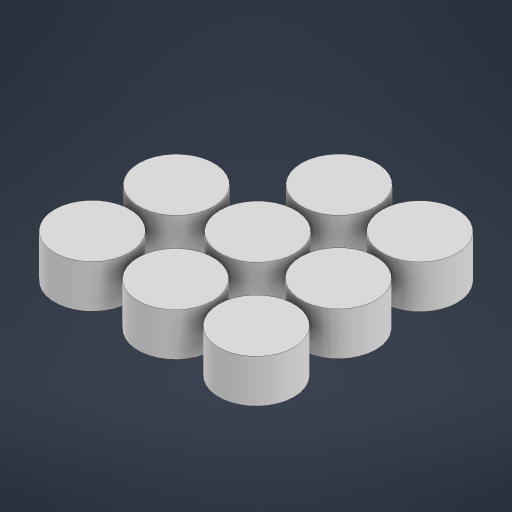
# Autodesk Inventor part: BUTTON
Saved by Autodesk Inventor 2024 (Build 280153000, 153)
## iProperties
Created: 2025-06-23
Part Number: BUTTON
Material: Generic
Document SubType Name: Modeling
Designer: ASUS
Density: 1 g/cm^3
Appearance: Default
Author: ASUS
Autodesk Inventor part; units mm, degrees
ref_plane "YZ Plane" through (0, 0, 0) normal (1, 0, 0) x (0, 1, 0)
ref_plane "XZ Plane" through (0, 0, 0) normal (0, 1, 0) x (-1, 0, 0)
ref_plane "XY Plane" through (0, 0, 0) normal (0, 0, 1) x (1, 0, 0)
sketch "Sketch1" plane through (0, 0, 0) normal (0, 1, 0) x (-1, 0, 0)
  circle A0 centre (0, 0) radius 7
  circle A1 centre (15.1273, 0) radius 7
  circle A2 centre (-15.0261, 0) radius 7
  circle A3 centre (0, -15.1556) radius 7
  circle A4 centre (0, 15.2765) radius 7
  circle A5 centre (-15.0261, 15.2765) radius 7
  circle A6 centre (15.5174, 15.2765) radius 7
  circle A7 centre (-15.0261, -15.1556) radius 7
  dimension "d0" = 14
  dimension "d1" = 14
  dimension "d2" = 14
  dimension "d3" = 14
  dimension "d4" = 14
  dimension "d5" = 14
  dimension "d6" = 14
  dimension "d7" = 14
  constraints: 8 centre point, 1 coincident
  measures "d0" diameter of A0
  measures "d1" diameter of A1
  measures "d2" diameter of A2
  measures "d3" diameter of A3
  measures "d4" diameter of A4
  measures "d5" diameter of A5
  measures "d6" diameter of A6
  measures "d7" diameter of A7
extrude "Extrusion1" add sketch "Sketch1" along normal blind 8
body "Solid1"
